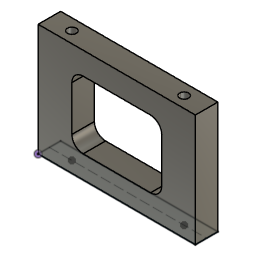
Wall_RPLidar (Autodesk Fusion 360 design; units mm, degrees)
Autodesk Fusion 360 part; units mm, degrees
note: some values were not read from the file. Set by a fixed rule: the direction of a hole.
sketch "Sketch1" plane through (0, 0, 0) normal (0, 0, 1) x (1, 0, 0)
  line L0 (0, 0) -> (70, 0)
  line L1 (70, 0) -> (70, 10)
  line L2 (70, 10) -> (0, 10)
  line L3 (0, 10) -> (0, 0)
  line L4 (0, 5) -> (70, 5) construction
  point P0 (10, 5)
  point P1 (60, 5)
  dimension "d1" = 70
  dimension "d2" = 10
  dimension "d9" = 50
  dimension "d10" = 10
  constraint horizontal L0
  constraint vertical L1
  constraint horizontal L2
  constraint vertical L3
  constraint coincident L0.start L3.end
  constraint midpoint L3 L4.start
  constraint midpoint L1 L4.end
  constraint coincident L4 P0
  constraint coincident L4 P1
  measures "d1" distance of L0.start L0.end
  measures "d2" distance of L0.start L2.end
  measures "d9" distance of P0 P1
  measures "d10" distance of L3 P0
extrude "Extrude1" add sketch "Sketch1" along normal blind 50
sketch "Sketch2" plane through (0, 0, 50) normal (0, 0, 1) x (-1, 0, 0)
  line L0 (0, -10) -> (0, 0)
  line L1 (0, 0) -> (-70, 0)
  line L2 (-70, 0) -> (-70, -10)
  line L3 (-70, -10) -> (0, -10)
  line L4 (0, -5) -> (-70, -5) construction
  line L5 (0, -10) -> (0, 0)
  point P0 (-10, -5)
  point P1 (-60, -5)
  dimension "d11" = 50
  dimension "d12" = 10
  constraint midpoint L0 L4.start
  constraint midpoint L2 L4.end
  constraint coincident L4 P0
  constraint coincident L4 P1
  measures "d11" distance of P0 P1
  measures "d12" distance of P0 L5
hole "Hole1" at (10, 5, 50) at (60, 5, 50) direction (0, 0, -1) diameter 4 depth 6 tip angle 180
hole "Hole2" at (10, 5, 0) at (60, 5, 0) direction (0, 0, 1) diameter 4 depth 6 tip angle 180
sketch "Sketch3" plane through (0, 0, 0) normal (0, -1, 0) x (1, 0, 0)
  line L0 (0, 0) -> (70, 0)
  line L1 (70, 0) -> (70, 50)
  line L2 (70, 50) -> (0, 50)
  line L3 (0, 50) -> (0, 0)
  line L4 (15, 40) -> (55, 40)
  line L5 (55, 40) -> (55, 10)
  line L6 (55, 10) -> (15, 10)
  line L7 (15, 10) -> (15, 40)
  line L8 (0, 0) -> (70, 0)
  dimension "d19" = 15
  dimension "d20" = 10
  dimension "d21" = 10
  dimension "d22" = 15
  constraint horizontal L4
  constraint vertical L5
  constraint horizontal L6
  constraint vertical L7
  measures "d19" distance of L3 L7
  measures "d20" distance of L2 L4
  measures "d21" distance of L6 L8
  measures "d22" distance of L1 L5
extrude "Extrude2" cut sketch "Sketch3" against normal blind 33 contours L4 L5 L6 L7
fillet "Fillet1" radius 5 4 edges at (15, 5, 40) (55, 5, 40) (55, 5, 10) (15, 5, 10)
equation "d10 = ( 70 mm - d9 ) / 2"
equation "d12 = ( 70 mm - d11 ) / 2"
